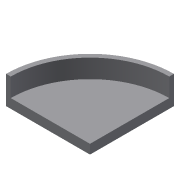
# Autodesk Inventor part: Chassis Piece 2
Saved by Autodesk Inventor 2017 (Build 210142000, 142)
## iProperties
Created: 2017-03-15
Part Number: Chassis Piece 2
Material: Generic
Document SubType Name: Modeling
Designer: zallen
Density: 1 g/cm^3
Appearance: Default
Author: zallen
Autodesk Inventor part; units mm, degrees
ref_plane "YZ Plane" through (0, 0, 0) normal (1, 0, 0) x (0, 1, 0)
ref_plane "XZ Plane" through (0, 0, 0) normal (0, 1, 0) x (-1, 0, 0)
ref_plane "XY Plane" through (0, 0, 0) normal (0, 0, 1) x (1, 0, 0)
sketch "Sketch1" plane through (0, 0, 0) normal (0, 1, 0) x (-1, 0, 0)
  circle A0 centre (0, 0) radius 228.6
  arc A1 (0, -228.6) -> (228.6, 0) centre (0, 0) ccw
  line L0 (228.6, 0) -> (0, 0)
  line L1 (0, 0) -> (0, -228.6)
  dimension "d0" = 457.2
  constraints: 4 end point, 4 point on circle, 2 centre point, 1 coincident, 1 concentric, 1 horizontal, 1 perpendicular
  measures "d0" diameter of A0
extrude "Extrusion1" add sketch "Sketch1" along normal blind 25.4 contours A0 L1 L0 picked at (152.0749, -7.0308)
sketch "Sketch2" plane through (0, 25.4, 0) normal (0, 1, 0) x (1, 0, 0)
  arc A0 (0, 228.6) -> (-228.6, 0) centre (0, 0) ccw projected
  arc A1 (0, 228.6) -> (-228.6, 0) centre (0, 0) ccw
  line L0 (-228.6, 0) -> (-215.9, 0)
  line L1 (-228.6, 0) -> (0, 0) projected
  line L2 (0, 228.6) -> (0, 215.9)
  line L3 (0, 0) -> (0, 228.6) projected
  arc A2 (0, 215.9) -> (-215.9, 0) centre (0, 0) ccw
  dimension "d6" = 12.7
  constraints: 4 end point, 4 point on circle, 2 centre point, 2 point on line, 1 concentric
  measures "d6" radial gap between concentric circles of A2 A0
extrude "Extrusion2" add sketch "Sketch2" along normal blind 50.8 contours L2 A2 L0 A0
body "Solid1"
